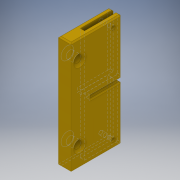
# Autodesk Inventor part: Aligner Helper v2
Saved by Autodesk Inventor 2019 (Build 230136000, 136)
## iProperties
Created: 2021-08-15
Part Number: Aligner Helper v2
Material: Generic
Document SubType Name: Modeling
Designer: Lix
Density: 1 g/cm^3
Appearance: Gold
Author: Lix
## iProperties of the stored document Aligner Helper v2_3DPrint.ipt
Created: 2021-08-20
Part Number: Aligner Helper v2_3DPrint
Material: Generic
Document SubType Name: Modeling
Designer: Lix
Density: 1 g/cm^3
Appearance: Default
Author: Lix
Autodesk Inventor part; units mm, degrees
ref_plane "YZ Plane" through (0, 0, 0) normal (1, 0, 0) x (0, 1, 0)
ref_plane "XZ Plane" through (0, 0, 0) normal (0, 1, 0) x (-1, 0, 0)
ref_plane "XY Plane" through (0, 0, 0) normal (0, 0, 1) x (1, 0, 0)
sketch "Sketch1" plane through (0, 0, 0) normal (0, 0, 1) x (1, 0, 0)
  line L0 (-5, 44.5) -> (5, 44.5)
  line L1 (5, 44.5) -> (5, -44.5)
  line L2 (5, -44.5) -> (-5, -44.5)
  line L3 (-5, -44.5) -> (-5, 44.5)
  line L4 (-5, 44.5) -> (5, -44.5) construction
  line L5 (5, 44.5) -> (-5, -44.5) construction
  point P0 (0, 0)
  dimension "d0" = 10
  dimension "d1" = 89
  constraints: 12 end point, 2 midpoint, 2 parallel, 1 horizontal, 1 perpendicular
  measures "d0" distance of L1.end L2.end
  measures "d1" distance of L0.end L1.end
extrude "Extrusion1" add sketch "Sketch1" along normal blind 40
sketch "Sketch2" plane through (0, 0, 0) normal (0, 0, -1) x (-1, 0, 0)
  line L0 (1.65, -44.5) -> (-1.65, -44.5)
  line L1 (-1.65, -44.5) -> (-1.65, 44.5)
  line L2 (-1.65, 44.5) -> (1.65, 44.5)
  line L3 (1.65, 44.5) -> (1.65, -44.5)
  line L4 (1.65, -44.5) -> (-1.65, 44.5) construction
  line L5 (-1.65, -44.5) -> (1.65, 44.5) construction
  line L6 (-5, -44.5) -> (5, -44.5) projected
  point P0 (0, 0)
  dimension "d4" = 3.3
  constraints: 12 end point, 2 midpoint, 2 parallel, 1 collinear, 1 horizontal, 1 perpendicular
  measures "d4" distance of L1.end L2.end
extrude "Extrusion2" cut sketch "Sketch2" against normal blind 26
sketch "Sketch4" plane through (5, -44.5, 0) normal (1, 0, 0) x (0, 0, -1)
  line L0 (-25, 42.9) -> (0, 42.9)
  line L1 (0, 42.9) -> (0, 46.1)
  line L2 (0, 46.1) -> (-25, 46.1)
  line L3 (-25, 46.1) -> (-25, 42.9)
  line L4 (0, 89) -> (0, 0) projected
  point P0 (0, 44.5)
  point P1 (0, 44.5)
  dimension "d15" = 25
  dimension "d16" = 3.2
  constraints: 8 end point, 2 midpoint, 2 parallel, 1 horizontal, 1 perpendicular
  measures "d15" distance of L2.end L1.end
  measures "d16" distance of L1.end L0.end
extrude "Extrusion3" cut sketch "Sketch4" against normal blind 16
sketch "Sketch3" plane through (5, -44.5, 0) normal (1, 0, 0) x (0, 0, -1)
  line L0 (0, 89) -> (-40, 89) projected
  line L1 (0, 89) -> (0, 0) projected
  line L2 (0, 0) -> (-40, 0) projected
  line L3 (-6.5, 5.9994) -> (-6.5, 83.0006) construction
  point P0 (0, 44.5)
  point P1 (-6.5, 44.5)
  point P2 (-26, 0)
  dimension "d19" = 19.5
  constraints: 2 coincident, 2 end point, 1 midpoint, 1 vertical
  measures "d19" distance from line of point (-26, 0) L3
hole "Hole1" at (5, 0, 6.5) at (5, -38.5006, 6.5) at (5, 38.5006, 6.5) direction (-1, 0, 0) diameter 3 depth 26.75
chamfer "Chamfer1" distance 1 angle 45 19 edges at (5, -44.5, 20) (-5, -44.5, 20) (5, 44.5, 20) (-5, 44.5, 20) (-3.325, -44.5, 0) (3.325, -44.5, 0) (-3.325, 44.5, 0) (3.325, 44.5, 0) (3.325, -1.6, 0) (3.325, 1.6, 0) (-3.325, 1.6, 0) (-3.325, -1.6, 0) (-5, -23.05, 0) (5, -1.6, 12.5) (5, -23.05, 0) (5, 23.05, 0) (-5, 23.05, 0) (0, 44.5, 40) (0, -44.5, 40)
sketch "Sketch5" plane through (5, -43.5, 40) normal (1, 0, 0) x (0, 0, -1)
  circle A0 centre (7, 14) radius 3
  line L0 (40, 0) -> (40, 40.9) projected
  line L1 (1, -1) -> (39, -1) projected
  circle A1 centre (7, 73) radius 3
  line L2 (39, 88) -> (1, 88) projected
  point P0 (40, 43.5)
  dimension "d23" = 6
  dimension "d24" = 33
  dimension "d25" = 15
  dimension "d26" = 15
  constraints: 2 centre point, 1 equal radius, 1 vertical alignment
  measures "d23" diameter of A0
  measures "d24" distance from line of A0.centre L0
  measures "d25" distance from line of A0.centre L1
  measures "d26" distance from line of A1.centre L2
extrude "Extrusion4" cut sketch "Sketch5" against normal blind 10
chamfer "Chamfer2" distance 2 angle 45 4 edges at (-5, -29.5, 36) (-5, 29.5, 36) (5, 29.5, 36) (5, -29.5, 36)
equation "\"d26\" = d25"
body "Solid1"
